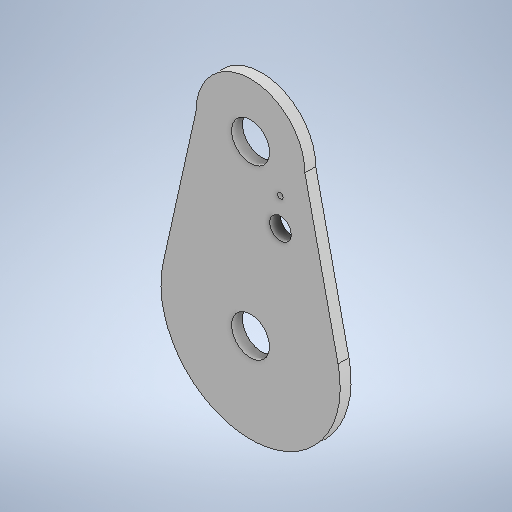
# Autodesk Inventor part: Placa de soporte
Saved by Autodesk Inventor 2025.3 (Build 293356030, 356C)
## iProperties
Created: 2025-08-24
Part Number: Placa de soporte
Material: Generic
Document SubType Name: Modeling
Designer: PC
Density: 1 g/cm^3
Appearance: Default
Author: PC
Autodesk Inventor part; units mm, degrees
ref_plane "YZ Plane" through (0, 0, 0) normal (1, 0, 0) x (0, 1, 0)
ref_plane "XZ Plane" through (0, 0, 0) normal (0, 1, 0) x (-1, 0, 0)
ref_plane "XY Plane" through (0, 0, 0) normal (0, 0, 1) x (1, 0, 0)
sketch "Sketch1" plane through (0, 0, 0) normal (0, 0, 1) x (1, 0, 0)
  arc A0 (-32.2108, 7.1739) -> (32.2108, 7.1739) centre (0, 0) ccw
  arc A1 (20, 62) -> (-20, 62) centre (0, 62) ccw
  line L0 (20, 62) -> (32.2108, 7.1739)
  line L1 (-20, 62) -> (-32.2108, 7.1739)
  circle A2 centre (0, 0) radius 7
  circle A3 centre (0, 62) radius 7
  circle A4 centre (11, 39.7881) radius 4
  circle A5 centre (11, 50.1761) radius 1
  dimension "d0" = 66
  dimension "d1" = 40
  dimension "d2" = 62
  dimension "d3" = 14
  dimension "d4" = 14
  dimension "d5" = 8
  dimension "d6" = 2
  dimension "d7" = 11
  constraints: 6 centre point, 4 end point, 4 point on circle, 3 coincident, 2 tangent, 1 vertical alignment
  measures "d0" diameter of A0
  measures "d1" diameter of A1
  measures "d2" distance of point (0, 0) A1.centre
  measures "d3" diameter of A2
  measures "d4" diameter of A3
  measures "d5" diameter of A4
  measures "d6" diameter of A5
  measures "d7" horizontal distance of A4.centre point (0, 0)
extrude "Extrusion1" add sketch "Sketch1" along normal blind 4
body "Solid1"
